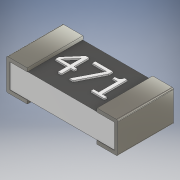
# Autodesk Inventor part: 21-1001
Saved by Autodesk Inventor 2018 (Build 220112000, 112)
## iProperties
Created: 2019-09-21
Part Number: 21-1001
Material: Copper
Document SubType Name: Modeling
Designer: Bradley
Density: 8.94 g/cm^3
Appearance: Smooth - White
Author: Bradley
Autodesk Inventor part; units mm, degrees
ref_plane "YZ Plane" through (0, 0, 0) normal (1, 0, 0) x (0, 1, 0)
ref_plane "XZ Plane" through (0, 0, 0) normal (0, 1, 0) x (-1, 0, 0)
ref_plane "XY Plane" through (0, 0, 0) normal (0, 0, 1) x (1, 0, 0)
sketch "Sketch1" plane through (0, 0, 0) normal (0, 1, 0) x (-1, 0, 0)
  line L0 (0.75, 0.175) -> (-0.75, 0.175)
  line L1 (-0.75, 0.175) -> (-0.75, -0.175)
  line L2 (-0.75, -0.175) -> (0.75, -0.175)
  line L3 (0.75, -0.175) -> (0.75, 0.175)
  line L4 (0.5, 0.175) -> (0.5, 0.225)
  line L5 (0.5, 0.225) -> (0.8, 0.225)
  line L6 (0.8, 0.225) -> (0.8, -0.225)
  line L7 (0.8, -0.225) -> (0.5, -0.225)
  line L8 (0.5, -0.225) -> (0.5, -0.175)
  line L9 (-0.5, 0.175) -> (-0.5, 0.225)
  line L10 (-0.5, 0.225) -> (-0.8, 0.225)
  line L11 (-0.8, 0.225) -> (-0.8, -0.225)
  line L12 (-0.8, -0.225) -> (-0.5, -0.225)
  line L13 (-0.5, -0.175) -> (-0.5, -0.225)
  line L14 (0.5, 0.175) -> (-0.5, 0.175)
  point P0 (0, 0)
  point P1 (0, 0.175)
  point P2 (0.75, 0)
  dimension "d0" = 1.6
  dimension "d1" = 0.05
  dimension "d2" = 0.05
  dimension "d3" = 0.45
  dimension "d4" = 0.3
  constraints: 30 end point, 12 point on line, 7 perpendicular, 3 collinear, 3 midpoint, 2 parallel, 1 horizontal, 1 horizontal alignment, 1 vertical, 1 vertical alignment
  measures "d0" distance between parallel lines of L11 L6
  measures "d1" distance of L7.end L8.end
  measures "d2" distance between parallel lines of L6 L3
  measures "d3" distance of L5.end L6.end
  measures "d4" distance of L6.end L7.end
extrude "Extrusion1" add sketch "Sketch1" along normal mid plane 0.8 contours L0 L4 L5 L6 L7 L8 L2 L3 | L0 L1 L2 L13 L12 L11 L10 L9
extrude "Extrusion2" add sketch "Sketch1" along normal mid plane 0.79 contours L3 L2 L1 L0
sketch "Sketch2" plane through (-0.5, -0.395, 0.175) normal (0, 0, 1) x (1, 0, 0)
  line L0 (0, 0) -> (0, 0.79) projected
  line L1 (1, 0) -> (0, 0) projected
  line L2 (1, 0) -> (1, 0.79) projected
  line L3 (0, 0.79) -> (1, 0.79) projected
  line L4 (0, 0.395) -> (1, 0.395) construction
  line L5 (0.3363, 0.3324) -> (0.2887, 0.3324)
  line L6 (0.2887, 0.3324) -> (0.2887, 0.195)
  line L7 (0.2887, 0.195) -> (0.2371, 0.195)
  line L8 (0.2371, 0.195) -> (0.2371, 0.3324)
  line L9 (0.2371, 0.3324) -> (0.0605, 0.3324)
  line L10 (0.0605, 0.3324) -> (0.0605, 0.3888)
  line L11 (0.0605, 0.3888) -> (0.2394, 0.595)
  line L12 (0.2394, 0.595) -> (0.2887, 0.595)
  line L13 (0.2887, 0.595) -> (0.2887, 0.3756)
  line L14 (0.2887, 0.3756) -> (0.3363, 0.3756)
  line L15 (0.3363, 0.3756) -> (0.3363, 0.3324)
  line L16 (0.2371, 0.3756) -> (0.2371, 0.5318)
  line L17 (0.2371, 0.5318) -> (0.1026, 0.3756)
  line L18 (0.1026, 0.3756) -> (0.2371, 0.3756)
  line L19 (0.6303, 0.535) -> (0.4572, 0.195)
  line L20 (0.4572, 0.195) -> (0.4002, 0.195)
  line L21 (0.4002, 0.195) -> (0.583, 0.548)
  line L22 (0.583, 0.548) -> (0.3765, 0.548)
  line L23 (0.3765, 0.548) -> (0.3765, 0.595)
  line L24 (0.3765, 0.595) -> (0.6303, 0.595)
  line L25 (0.6303, 0.595) -> (0.6303, 0.535)
  line L26 (0.9058, 0.195) -> (0.7107, 0.195)
  line L27 (0.7107, 0.195) -> (0.7107, 0.2358)
  line L28 (0.7107, 0.2358) -> (0.7833, 0.2358)
  line L29 (0.7833, 0.2358) -> (0.7833, 0.5039)
  line L30 (0.7833, 0.5039) -> (0.7107, 0.5039)
  line L31 (0.7107, 0.5039) -> (0.7107, 0.5405)
  spline S0 degree 2 poles (0.7107, 0.5405) (0.7519, 0.5405) (0.7908, 0.5639) (0.7934, 0.5963) knots 0 0 0 1 2 2 2
  line L32 (0.7934, 0.5963) -> (0.8348, 0.5963)
  line L33 (0.8348, 0.5963) -> (0.8348, 0.2358)
  line L34 (0.8348, 0.2358) -> (0.9058, 0.2358)
  line L35 (0.9058, 0.2358) -> (0.9058, 0.195)
  point P0 (0.5, 0.395)
  constraints: 2 end point, 2 midpoint, 1 horizontal
extrude "Extrusion3" add sketch "Sketch2" along normal blind 0.02 contours L5 L6 L7 L8 L9 L10 L11 L12 L13 L14 L15 | L19 L20 L21 L22 L23 L24 L25 | L26 L27 L28 L29 L30 L31 S0 L32 L33 L34 L35
fillet "Fillet1" radius 0.02 4 edges at (-0.8, 0, 0.225) (-0.8, 0, -0.225) (0.8, 0, 0.225) (0.8, 0, -0.225)
equation "\"d2\" = d1"
body "Solid1"
